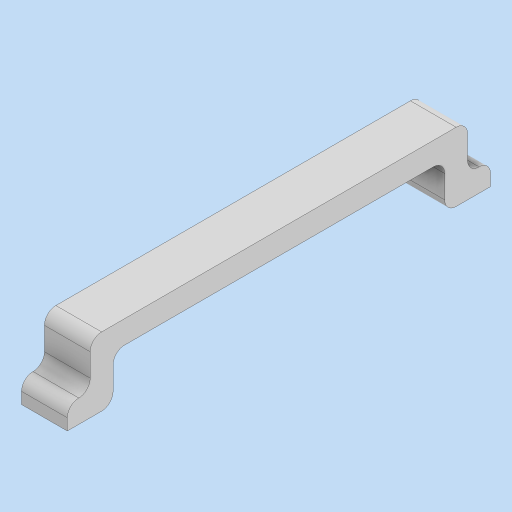
# Autodesk Inventor part: screen_support
Saved by Autodesk Inventor 2024 (Build 280153000, 153)
## iProperties
Created: 2024-05-14
Part Number: screen_support
Material: Generic
Document SubType Name: Modeling
Designer: fredyespana
Density: 1 g/cm^3
Appearance: Default
Author: fredyespana
Autodesk Inventor part; units mm, degrees
ref_plane "YZ Plane" through (0, 0, 0) normal (1, 0, 0) x (0, 1, 0)
ref_plane "XZ Plane" through (0, 0, 0) normal (0, 1, 0) x (-1, 0, 0)
ref_plane "XY Plane" through (0, 0, 0) normal (0, 0, 1) x (1, 0, 0)
sketch "Sketch1" plane through (0, 0, 0) normal (0, 1, 0) x (-1, 0, 0)
  line L0 (0, 18.5) -> (4, 18.5)
  line L1 (4, 18.5) -> (4, 14.5)
  line L2 (4, 14.5) -> (0, 14.5)
  line L3 (0, 14.5) -> (0, 18.5)
  line L4 (4, -14.5) -> (0, -14.5)
  line L5 (0, -14.5) -> (0, -18.5)
  line L6 (0, -18.5) -> (4, -18.5)
  line L7 (4, -18.5) -> (4, -14.5)
  line L8 (4, 14.5) -> (4, -14.5) construction
  point P0 (0, 0)
  point P1 (4, 0)
  dimension "d0" = 37
  dimension "d1" = 4
  constraints: 18 end point, 4 parallel, 3 equal length, 2 horizontal, 2 perpendicular, 1 horizontal alignment, 1 midpoint, 1 point on line, 1 vertical, 1 vertical alignment
  measures "d0" distance between parallel lines of L6 L0
  measures "d1" distance of L5.end L6.end
extrude "Extrusion1" add sketch "Sketch1" along normal blind 2
sketch "Sketch2" plane through (0, 2, 0) normal (0, 1, 0) x (1, 0, 0)
  line L0 (-4, -14.5) -> (-4, -18.5) projected
  line L1 (0, 14.5) -> (0, 18.5) projected
  line L2 (-4, -16.5) -> (0, -16.5)
  line L3 (0, -16.5) -> (0, 16.5)
  line L4 (0, 16.5) -> (-4, 16.5)
  line L5 (-4, 16.5) -> (-4, -16.5)
  line L6 (0, -14.5) -> (-4, -14.5) projected
  line L7 (-4, 14.5) -> (0, 14.5) projected
  point P0 (0, 0)
  dimension "d4" = 2
  dimension "d5" = 2
  constraints: 8 end point, 2 midpoint, 2 parallel, 1 horizontal, 1 perpendicular
  measures "d4" distance between parallel lines of L2 L6
  measures "d5" distance between parallel lines of L4 L7
extrude "Extrusion2" add sketch "Sketch2" along normal blind 2 contours L6 L3 L2 L0 | L5 L4 L1 L7
sketch "Sketch3" plane through (0, 4, 0) normal (0, 1, 0) x (1, 0, 0)
  line L0 (-4, -16.5) -> (0, -16.5) projected
  line L1 (0, 16.5) -> (-4, 16.5) projected
  line L2 (0, -16.5) -> (-4, -16.5)
  line L3 (-4, -16.5) -> (-4, 16.5)
  line L4 (-4, 16.5) -> (0, 16.5)
  line L5 (0, 16.5) -> (0, -16.5)
  point P0 (0, 0)
  constraints: 8 end point, 2 parallel, 1 horizontal, 1 perpendicular
extrude "Extrusion3" add sketch "Sketch3" along normal blind 2
fillet "Fillet3" radius 1 9 edges at (-2, 2, 16.5) (-2, 2, 18.5) (-2, 2, -16.5) (-2, 0, 14.5) (-2, 0, -14.5) (-2, 4, -14.5) (-2, 4, 14.5) (-2, 6, -16.5) (-2, 6, 16.5)
fillet "Fillet4" radius 1 1 edges at (-2, 2, -18.5)
body "Solid1"
